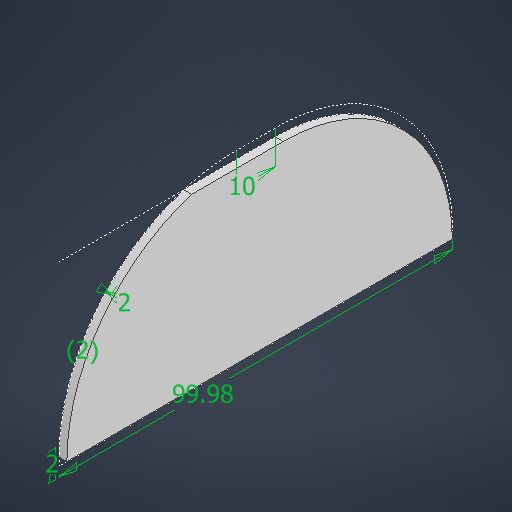
# Autodesk Inventor part: BuddyRobotBaseDoor
Saved by Autodesk Inventor 2026.2 (Build 302298000, 298)
## iProperties
Created: 2026-09-15
Part Number: BuddyRobotBaseDoor
Material: Generic
Document SubType Name: Modeling
Designer: User
Density: 1 g/cm^3
Appearance: Default
Author: User
Autodesk Inventor part; units mm, degrees
ref_plane "YZ Plane" through (0, 0, 0) normal (1, 0, 0) x (0, 1, 0)
ref_plane "XZ Plane" through (0, 0, 0) normal (0, 1, 0) x (-1, 0, 0)
ref_plane "XY Plane" through (0, 0, 0) normal (0, 0, 1) x (1, 0, 0)
sketch "Sketch1" plane through (0, 0, 0) normal (1, 0, 0) x (0, 1, 0)
  line L0 (0, 49.99) -> (2, 49.99) construction
  line L1 (2, 49.99) -> (2, -49.99) construction
  line L2 (2, -49.99) -> (0, -49.99) construction
  line L3 (0, 49.99) -> (0, 0) construction
  line L4 (0, 0) -> (0, -49.99) construction
  arc A0 (46.99, 5) -> (2, 49.99) centre (2, 5) ccw construction
  arc A1 (2, -49.99) -> (46.99, -5) centre (2, -5) ccw construction
  line L5 (46.99, 5) -> (46.99, -5) construction
  arc A2 (2, -47.99) -> (44.99, -5) centre (2, -5) ccw construction
  line L6 (44.99, -5) -> (44.99, 5) construction
  arc A3 (44.99, 5) -> (2, 47.99) centre (2, 5) ccw construction
  line L7 (44.99, 5) -> (44.99, 49.99) construction
  dimension "d0" = 99.98
  dimension "d1" = 2
  dimension "d2" = 10
  dimension "d3" = 2
  dimension "d4" = 2
  constraints: 16 end point, 8 point on circle, 4 centre point, 4 tangent, 4 vertical, 2 perpendicular, 2 point on line, 1 collinear, 1 equal radius, 1 horizontal, 1 horizontal alignment, 1 vertical alignment, 2 other
  measures "d0" distance of L0.start L2.end
  measures "d1" distance of L0.start L0.end
  measures "d2" distance of L5.start L5.end
  measures "d3" radial gap between concentric circles of A0 A3
  measures "d4" radial gap between concentric circles of A0 A3
sketch "Sketch2" plane through (0, 0, 0) normal (1, 0, 0) x (0, 1, 0)
  line L0 (0, 49.99) -> (2, 49.99) construction
  line L1 (2, 49.99) -> (2, -49.99) construction
  line L2 (2, -49.99) -> (0, -49.99) construction
  line L3 (0, 49.99) -> (0, 0) construction
  line L4 (0, 0) -> (0, -49.99) construction
  arc A0 (46.99, 5) -> (2, 49.99) centre (2, 5) ccw construction
  arc A1 (2, -49.99) -> (46.99, -5) centre (2, -5) ccw construction
  line L5 (46.99, 5) -> (46.99, -5) construction
  arc A2 (2, -47.99) -> (44.99, -5) centre (2, -5) ccw construction
  line L6 (44.99, -5) -> (44.99, 5) construction
  arc A3 (44.99, 5) -> (2, 47.99) centre (2, 5) ccw construction
  line L7 (44.99, 5) -> (44.99, 49.99) construction
  line L8 (2, 49.99) -> (2, -47.99)
  arc A4 (2, -47.99) -> (44.99, -5) centre (2, -5) ccw
  line L9 (44.99, -5) -> (44.99, 18.265)
  arc A5 (44.99, 18.265) -> (2, 49.99) centre (2, 5) ccw
  constraints: 6 point on circle, 4 end point, 3 concentric, 2 centre point, 2 point on line, 1 collinear
extrude "Extrusion1" add sketch "Sketch2" along normal blind 1.98
sketch "Sketch3" plane through (0, 0, 0) normal (-1, 0, 0) x (0, 0, 1)
  line L0 (26.265, 33.495) -> (26.265, 13.495)
  arc A0 (26.265, 13.495) -> (26.265, 33.495) centre (26.265, 23.495) ccw
  line L1 (-5, 44.99) -> (18.265, 44.99) projected
  line L2 (18.265, 44.99) -> (18.265, 23.495)
  line L3 (18.265, 23.495) -> (18.265, 2)
  line L4 (49.99, 2) -> (-47.99, 2) projected
  point P0 (0, 0)
  dimension "d7" = 20
  dimension "d8" = 8
  constraints: 6 end point, 2 point on circle, 2 point on line, 2 vertical, 1 centre point, 1 collinear, 1 horizontal alignment, 1 midpoint
  measures "d7" distance of L0.start L0.end
  measures "d8" distance between parallel lines of L0 L3
extrude "Extrusion2" cut sketch "Sketch3" against normal blind 1
fillet "Fillet1" radius 2 1 edges at (0, 23.495, 36.265)
body "Solid1"
